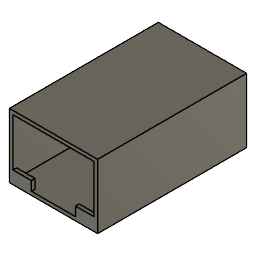
holder_bracket (Autodesk Fusion 360 design; units mm, degrees)
part number: 2025-11-27-19-42-51-452
part number: 2025-11-29-21-01-25-605
Autodesk Fusion 360 part; units mm, degrees
note: some values were not read from the file. Set by a fixed rule: which sketch regions a step uses.
sketch "Szkic1" plane through (0, 0, 0) normal (0, 0, 1) x (1, 0, 0)
  line L0 (0, 0) -> (48, 0)
  line L1 (48, 0) -> (48, 81)
  line L2 (48, 81) -> (0, 81)
  line L3 (0, 81) -> (0, 0)
  dimension "d1" = 48
  dimension "d2" = 81
  constraint horizontal L0
  constraint vertical L1
  constraint horizontal L2
  constraint vertical L3
  constraint coincident L0.start L3.end
  measures "d1" distance of L0.start L0.end
  measures "d2" distance of L0.start L2.end
extrude "Wyciągnięcie proste1" add sketch "Szkic1" along normal blind 2 makes body 1
ref_plane "Płaszczyzna konstrukcyjna1" through (0, 0, 2) normal (0, 0, 1) x (1, 0, 0)
sketch "Szkic2" plane through (0, 0, 2) normal (0, 0, 1) x (1, 0, 0)
  line L0 (0, 2) -> (2, 2) construction
  line L1 (0, 0) -> (48, 0)
  line L2 (48, 0) -> (48, 81)
  line L3 (48, 81) -> (0, 81)
  line L4 (0, 81) -> (0, 0)
  line L5 (2, 2) -> (12, 2)
  line L6 (12, 2) -> (12, 0)
  line L7 (12, 0) -> (2, 0)
  line L8 (2, 0) -> (2, 2)
  line L9 (46, 2) -> (36, 2)
  line L10 (36, 2) -> (36, 0)
  line L11 (36, 0) -> (46, 0)
  line L12 (46, 0) -> (46, 2)
  line L13 (0, 0) -> (2, 0)
  line L14 (2, 0) -> (2, 81)
  line L15 (2, 81) -> (0, 81)
  line L16 (0, 81) -> (0, 0)
  line L17 (48, 0) -> (46, 0)
  line L18 (46, 0) -> (46, 81)
  line L19 (46, 81) -> (48, 81)
  line L20 (48, 81) -> (48, 0)
  dimension "d8" = 44
  dimension "d10" = 48
  dimension "d11" = 81
  dimension "d12" = 10
  dimension "d13" = 2
  dimension "d16" = 10
  dimension "d19" = 81
  dimension "d22" = 81
  constraint horizontal L1
  constraint vertical L2
  constraint horizontal L3
  constraint vertical L4
  constraint coincident L1.start L4.end
  constraint horizontal L5
  constraint vertical L6
  constraint horizontal L7
  constraint vertical L8
  constraint horizontal L9
  constraint vertical L10
  constraint horizontal L11
  constraint vertical L12
  constraint horizontal L13
  constraint vertical L14
  constraint horizontal L15
  constraint vertical L16
  constraint horizontal L17
  constraint vertical L18
  constraint horizontal L19
  constraint vertical L20
  measures "d8" distance of L0.end L9.start
  measures "d10" distance of L1.start L1.end
  measures "d11" distance of L1.start L3.end
  measures "d12" distance of L0.end L5.end
  measures "d13" distance of L0.end L7.end
  measures "d16" distance of L9.start L9.end
  measures "d19" distance of L1.start L3.end
  measures "d22" distance of L1.end L2.end
extrude "Wyciągnięcie proste2" add sketch "Szkic2" along normal blind 5 contours L1 L5 L6 L7 L8 L14 bodies 1
extrude "Wyciągnięcie proste3" add sketch "Szkic2" along normal blind 5 contours L1 L9 L10 L11 L12 L18 bodies 1
extrude "Wyciągnięcie proste4" add sketch "Szkic2" along normal blind 31 contours L1 L3 L4 L8 L13 L14 L15 L16 bodies 1
extrude "Wyciągnięcie proste5" add sketch "Szkic2" along normal blind 31 contours L1 L2 L3 L12 L17 L18 L19 L20 bodies 1
ref_plane "Płaszczyzna konstrukcyjna2" through (0, 0, 33) normal (0, 0, 1) x (1, 0, 0)
sketch "Szkic3" plane through (0, 0, 33) normal (0, 0, 1) x (1, 0, 0)
  line L0 (0, 0) -> (48, 0)
  line L1 (48, 0) -> (48, 81)
  line L2 (48, 81) -> (0, 81)
  line L3 (0, 81) -> (0, 0)
  dimension "d26" = 48
  dimension "d27" = 81
  constraint horizontal L0
  constraint vertical L1
  constraint horizontal L2
  constraint vertical L3
  constraint coincident L0.start L3.end
  measures "d26" distance of L0.start L0.end
  measures "d27" distance of L0.start L2.end
extrude "Wyciągnięcie proste6" add sketch "Szkic3" along normal blind 2 bodies 1
copy_body "Bryła->Komponent1" bodies 1 removing the originals makes body 2 in component "Component"
component "Component" placed x (1, 0, 0) y (0, 1, 0) z (0, 0, 1) at (0, 0, 0)
